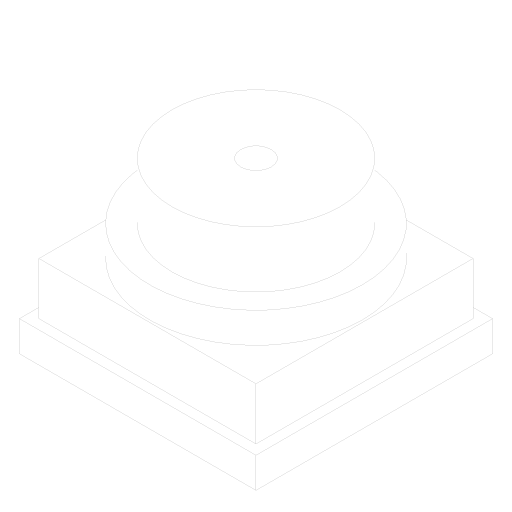
# Autodesk Inventor part: Camera
Saved by Autodesk Inventor 2023 (Build 270158000, 158)
## iProperties
Created: 2024-03-21
Part Number: Camera
Material: Generic
Document SubType Name: Modeling
Designer: ferrerx
Density: 1 g/cm^3
Appearance: Glossy - Black
Author: ferrerx
Autodesk Inventor part; units mm, degrees
ref_plane "YZ Plane" through (0, 0, 0) normal (1, 0, 0) x (0, 1, 0)
ref_plane "XZ Plane" through (0, 0, 0) normal (0, 1, 0) x (-1, 0, 0)
ref_plane "XY Plane" through (0, 0, 0) normal (0, 0, 1) x (1, 0, 0)
sketch "Sketch1" plane through (0, 0, 0) normal (0, 1, 0) x (-1, 0, 0)
  circle A0 centre (0, 0) radius 1.935
  dimension "d0" = 3.87
  constraints: 1 centre point, 1 coincident
  measures "d0" diameter of A0
extrude "Extrusion1" add sketch "Sketch1" along normal blind 2
sketch "Sketch2" plane through (0, 0, 0) normal (0, -1, 0) x (1, 0, 0)
  line L0 (2.5, 2.5) -> (-2.5, 2.5)
  line L1 (-2.5, 2.5) -> (-2.5, -2.5)
  line L2 (-2.5, -2.5) -> (2.5, -2.5)
  line L3 (2.5, -2.5) -> (2.5, 2.5)
  line L4 (2.5, 2.5) -> (-2.5, -2.5) construction
  line L5 (-2.5, 2.5) -> (2.5, -2.5) construction
  point P0 (0, 0)
  dimension "d9" = 5
  dimension "d10" = 5
  constraints: 12 end point, 2 midpoint, 2 parallel, 1 horizontal, 1 perpendicular
  measures "d9" distance of L1.end L2.end
  measures "d10" distance of L0.end L1.end
extrude "Extrusion2" add sketch "Sketch2" along normal blind 1.2
sketch "Sketch3" plane through (0, -1.2, 0) normal (0, -1, 0) x (1, 0, 0)
  line L0 (2.725, 2.725) -> (-2.725, 2.725)
  line L1 (-2.725, 2.725) -> (-2.725, -2.725)
  line L2 (-2.725, -2.725) -> (2.725, -2.725)
  line L3 (2.725, -2.725) -> (2.725, 2.725)
  line L4 (2.725, 2.725) -> (-2.725, -2.725) construction
  line L5 (-2.725, 2.725) -> (2.725, -2.725) construction
  point P0 (0, 0)
  dimension "d5" = 5.45
  dimension "d6" = 5.45
  constraints: 12 end point, 2 midpoint, 2 parallel, 1 horizontal, 1 perpendicular
  measures "d5" distance of L0.end L1.end
  measures "d6" distance of L1.end L2.end
extrude "Extrusion3" add sketch "Sketch3" along normal blind 0.7
sketch "Sketch4" plane through (0, 0, 0) normal (0, 1, 0) x (1, 0, 0)
  circle A0 centre (0, 0) radius 2.45
  dimension "d11" = 4.9
  constraints: 1 centre point, 1 coincident
  measures "d11" diameter of A0
extrude "Extrusion4" add sketch "Sketch4" along normal blind 0.7
sketch "Sketch5" plane through (0, 2, 0) normal (0, 1, 0) x (1, 0, 0)
  circle A0 centre (0, 0) radius 0.35
  dimension "d14" = 0.7
  constraints: 1 centre point, 1 coincident
  measures "d14" diameter of A0
extrude "Extrusion5" cut sketch "Sketch5" against normal blind 0.7
body "Solid1"
